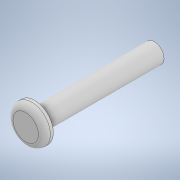
# Autodesk Inventor part: m0.6screw_4mm
Saved by Autodesk Inventor 2021 (Build 250183000, 183)
## iProperties
Created: 2022-02-03
Part Number: m0.6screw_4mm
Material: Generic
Document SubType Name: Sheet Metal
Designer: Unit-005
Density: 1 g/cm^3
Sheet Metal Rule: Default
Appearance: Default
Author: Unit-005
Autodesk Inventor part; units mm, degrees
ref_plane "YZ Plane" through (0, 0, 0) normal (1, 0, 0) x (0, 1, 0)
ref_plane "XZ Plane" through (0, 0, 0) normal (0, 1, 0) x (-1, 0, 0)
ref_plane "XY Plane" through (0, 0, 0) normal (0, 0, 1) x (1, 0, 0)
sketch "Sketch2" plane through (0, 0, 0) normal (1, 0, 0) x (0, 1, 0)
  line L0 (0, 3.16) -> (0, -2.86) projected
  line L1 (-0.875, 0) -> (0.875, 0) projected
  line L2 (0.325, 2) -> (-0.325, 2)
  line L3 (-0.325, 2) -> (-0.325, -2)
  line L4 (-0.325, -2) -> (0.325, -2)
  line L5 (0.325, -2) -> (0.325, 2)
  line L6 (0.325, 2) -> (-0.325, -2) construction
  line L7 (-0.325, 2) -> (0.325, -2) construction
  line L8 (0.625, 2) -> (-0.625, 2)
  line L9 (-0.625, 2) -> (-0.625, 2.3)
  line L10 (-0.625, 2.3) -> (0.625, 2.3)
  line L11 (0.625, 2.3) -> (0.625, 2)
  point P0 (0, 0)
  point P1 (0, 2)
  point P2 (0, 2.3)
  point P3 (0, -2)
  dimension "d0" = 0.65
  dimension "d1" = 4
  dimension "d2" = 1.25
  dimension "d3" = 0.3
  constraints: 20 end point, 4 midpoint, 4 parallel, 2 horizontal, 2 perpendicular, 1 point on line
  measures "d0" distance of L4.end L3.end
  measures "d1" distance of L3.end L2.end
  measures "d2" distance of L9.end L10.end
  measures "d3" distance of L8.end L9.end
revolve "Revolution1" add sketch "Sketch2" angle 360 about axis through (0, 0, 0) along (0, 0, -1) contours L10 L11 L8 L2 L0 | L2 L5 L1 L0 | L1 L5 L4 L0
fillet "Fillet1" radius 0.2 1 edges at (0, -0.625, 2.3)
equation "\"BendRadius\" = Thickness"
equation "\"BendReliefWidth\" = Thickness"
equation "\"BendReliefDepth\" = 0.5 * Thickness"
equation "\"CornerReliefSize\" = 4 * Thickness"
equation "\"MinimumRemnant\" = 2 * Thickness"
equation "\"TransitionRadius\" = BendRadius"
equation "\"JacobiRadiusSize\" = BendRadius"
equation "\"GapSize\" = Thickness"
equation "\"Thickness\" = 3.048"
body "Solid1"
